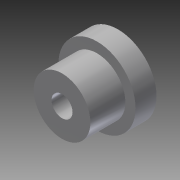
# Autodesk Inventor part: 10 th sprocket
Saved by Autodesk Inventor 2014 SP1 (Build 180222100, 222)
## iProperties
Created: 2014-02-21
Part Number: 10 th sprocket
Material: Steel
Document SubType Name: Modeling
Designer: Asif
Mass: 122.766 g
Surface Area: 48.7733 cm^2
Volume: 15.639 cm^3
Density: 7.85 g/cm^3
Appearance: Steel
Author: Asif
Autodesk Inventor part; units mm, degrees
ref_plane "YZ Plane" through (0, 0, 0) normal (1, 0, 0) x (0, 1, 0)
ref_plane "XZ Plane" through (0, 0, 0) normal (0, 1, 0) x (-1, 0, 0)
ref_plane "XY Plane" through (0, 0, 0) normal (0, 0, 1) x (1, 0, 0)
sketch "Sketch1" plane through (0, 0, 0) normal (0, 0, 1) x (1, 0, 0)
  circle A0 centre (0, 0) radius 17.5133
  circle A1 centre (0, 0) radius 4.7625
  dimension "d0" = 35.0266
  dimension "d1" = 9.525
  constraints: 2 centre point, 2 coincident
  measures "d0" diameter of A0
  measures "d1" diameter of A1
extrude "Extrusion1" add sketch "Sketch1" along normal blind 25.4
sketch "Sketch2" plane through (0, 0, 25.4) normal (0, 0, 1) x (1, 0, 0)
  circle A0 centre (0, 0) radius 17.5133 projected
  circle A1 centre (0, 0) radius 12.8778
  dimension "d4" = 25.7556
  constraints: 1 centre point, 1 coincident
  measures "d4" diameter of A1
extrude "Extrusion2" cut sketch "Sketch2" against normal blind 15.875
body "Solid1"
